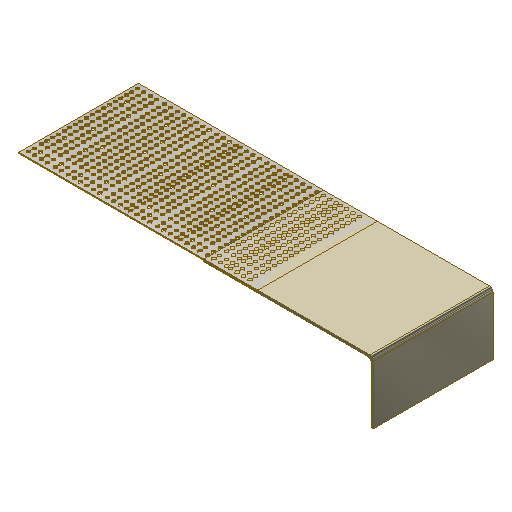
# Autodesk Inventor part: eletrodo - nickel e titanio
Saved by Autodesk Inventor 2025 (Build 290162000, 162)
## iProperties
Created: 2024-12-11
Part Number: eletrodo - nickel e titanio
Material: Genérico
Document SubType Name: Modeling
Designer: November
Density: 1 g/cm^3
Appearance: Padrão
Author: November
Autodesk Inventor part; units mm, degrees
(part 1 of 4)
ref_plane "YZ Plane" through (0, 0, 0) normal (1, 0, 0) x (0, 1, 0)
ref_plane "XZ Plane" through (0, 0, 0) normal (0, 1, 0) x (-1, 0, 0)
ref_plane "XY Plane" through (0, 0, 0) normal (0, 0, 1) x (1, 0, 0)
sketch "Esboço1" plane through (0, 0, 0) normal (0, 0, 1) x (1, 0, 0)
  line L0 (0, 0) -> (0, 5)
  line L1 (0, 5) -> (-14, 5)
  line L2 (0, 0) -> (0.2, 0)
  line L3 (0.2, 0) -> (0.2, 5.2)
  line L4 (-14, 5) -> (-14, 5.2)
  line L5 (-14, 5.2) -> (0.2, 5.2)
  dimension "d0" = 5
  dimension "d1" = 14
  dimension "d2" = 0.2
  dimension "d3" = 5.2
  dimension "d4" = 0.2
  constraints: 12 end point, 2 horizontal, 2 perpendicular, 2 vertical, 1 point on line
  measures "d0" distance of L0.start L0.end
  measures "d1" distance of L0.end L1.end
  measures "d2" distance of L0.start L2.end
  measures "d3" distance of L2.end L3.end
  measures "d4" distance of L1.end L4.end
extrude "Extrusão1" add sketch "Esboço1" along normal blind 10
fillet "Arredondamento1" radius 0.3 1 edges at (0.2, 5.2, 5)
fillet "Arredondamento2" radius 0.3 1 edges at (0, 5, 5)
sketch "Esboço2" plane through (-14, 5.2, 10) normal (0, 1, 0) x (1, 0, 0)
  line L0 (0, 10) -> (13.7, 10)
  line L1 (4.5193, 10) -> (-15.4807, 10)
  line L2 (-15.4807, 10) -> (-15.4807, 0)
  line L3 (-15.4807, 0) -> (4.5193, 0)
  line L4 (4.5193, 0) -> (4.5193, 10)
  point P0 (14, 10)
  point P1 (-5.4807, 0)
  dimension "d9" = 20
  dimension "d10" = 10
  constraints: 8 end point, 2 parallel, 1 horizontal, 1 midpoint, 1 perpendicular, 1 point on line
  measures "d9" distance of L3.end L2.end
  measures "d10" distance from line of point (-5.481, 0) L1
extrude "Extrusão2" add sketch "Esboço2" against normal blind 0.1 separate body
sketch "Esboço3" plane through (-14, 5.2, 10) normal (0, 1, 0) x (1, 0, 0)
  line L0 (-15.1346, 9.764) -> (-15.3015, 9.5833)
  line L1 (-15.3015, 9.5833) -> (-15.1346, 9.3971)
  line L2 (-15.1346, 9.764) -> (-14.9676, 9.5833)
  line L3 (-14.9676, 9.5833) -> (-15.1346, 9.3971)
  line L4 (-15.1346, 9.2863) -> (-15.3015, 9.1056)
  line L5 (-15.3015, 9.1056) -> (-15.1346, 8.9195)
  line L6 (-15.1346, 9.2863) -> (-14.9676, 9.1056)
  line L7 (-14.9676, 9.1056) -> (-15.1346, 8.9195)
  line L8 (-15.1346, 8.827) -> (-15.3015, 8.6463)
  line L9 (-15.3015, 8.6463) -> (-15.1346, 8.4602)
  line L10 (-15.1346, 8.827) -> (-14.9676, 8.6463)
  line L11 (-14.9676, 8.6463) -> (-15.1346, 8.4602)
  line L12 (-15.1346, 8.3637) -> (-15.3015, 8.183)
  line L13 (-15.3015, 8.183) -> (-15.1346, 7.9969)
  line L14 (-15.1346, 8.3637) -> (-14.9676, 8.183)
  line L15 (-14.9676, 8.183) -> (-15.1346, 7.9969)
  line L16 (-15.1346, 7.8983) -> (-15.3015, 7.7177)
  line L17 (-15.3015, 7.7177) -> (-15.1346, 7.5315)
  line L18 (-15.1346, 7.8983) -> (-14.9676, 7.7177)
  line L19 (-14.9676, 7.7177) -> (-15.1346, 7.5315)
  line L20 (-15.1346, 7.4088) -> (-15.3015, 7.2281)
  line L21 (-15.3015, 7.2281) -> (-15.1346, 7.042)
  line L22 (-15.1346, 7.4088) -> (-14.9676, 7.2281)
  line L23 (-14.9676, 7.2281) -> (-15.1346, 7.042)
  line L24 (-15.1346, 6.9434) -> (-15.3015, 6.7628)
  line L25 (-15.3015, 6.7628) -> (-15.1346, 6.5766)
  line L26 (-15.1346, 6.9434) -> (-14.9676, 6.7628)
  line L27 (-14.9676, 6.7628) -> (-15.1346, 6.5766)
  line L28 (-15.1346, 6.4539) -> (-15.3015, 6.2732)
  line L29 (-15.3015, 6.2732) -> (-15.1346, 6.0871)
  line L30 (-15.1346, 6.4539) -> (-14.9676, 6.2732)
  line L31 (-14.9676, 6.2732) -> (-15.1346, 6.0871)
  line L32 (-15.1346, 5.9825) -> (-15.3015, 5.8018)
  line L33 (-15.3015, 5.8018) -> (-15.1346, 5.6157)
  line L34 (-15.1346, 5.9825) -> (-14.9676, 5.8018)
  line L35 (-14.9676, 5.8018) -> (-15.1346, 5.6157)
  line L36 (-15.1346, 5.4909) -> (-15.3015, 5.3102)
  line L37 (-15.3015, 5.3102) -> (-15.1346, 5.124)
  line L38 (-15.1346, 5.4909) -> (-14.9676, 5.3102)
  line L39 (-14.9676, 5.3102) -> (-15.1346, 5.124)
  line L40 (-15.1346, 5.0132) -> (-15.3015, 4.8325)
  line L41 (-15.3015, 4.8325) -> (-15.1346, 4.6463)
  line L42 (-15.1346, 5.0132) -> (-14.9676, 4.8325)
  line L43 (-14.9676, 4.8325) -> (-15.1346, 4.6463)
  line L44 (-15.1346, 4.5539) -> (-15.3015, 4.3732)
  line L45 (-15.3015, 4.3732) -> (-15.1346, 4.187)
  line L46 (-15.1346, 4.5539) -> (-14.9676, 4.3732)
  line L47 (-14.9676, 4.3732) -> (-15.1346, 4.187)
  line L48 (-15.1346, 4.0906) -> (-15.3015, 3.9099)
  line L49 (-15.3015, 3.9099) -> (-15.1346, 3.7237)
  line L50 (-15.1346, 4.0906) -> (-14.9676, 3.9099)
  line L51 (-14.9676, 3.9099) -> (-15.1346, 3.7237)
  line L52 (-15.1346, 3.6252) -> (-15.3015, 3.4445)
  line L53 (-15.3015, 3.4445) -> (-15.1346, 3.2584)
  line L54 (-15.1346, 3.6252) -> (-14.9676, 3.4445)
  line L55 (-14.9676, 3.4445) -> (-15.1346, 3.2584)
  line L56 (-15.1346, 3.1357) -> (-15.3015, 2.955)
  line L57 (-15.3015, 2.955) -> (-15.1346, 2.7688)
  line L58 (-15.1346, 3.1357) -> (-14.9676, 2.955)
  line L59 (-14.9676, 2.955) -> (-15.1346, 2.7688)
  line L60 (-15.1346, 2.6703) -> (-15.3015, 2.4896)
  line L61 (-15.3015, 2.4896) -> (-15.1346, 2.3035)
  line L62 (-15.1346, 2.6703) -> (-14.9676, 2.4896)
  line L63 (-14.9676, 2.4896) -> (-15.1346, 2.3035)
  line L64 (-15.1346, 2.1808) -> (-15.3015, 2.0001)
  line L65 (-15.3015, 2.0001) -> (-15.1346, 1.8139)
  line L66 (-15.1346, 2.1808) -> (-14.9676, 2.0001)
  line L67 (-14.9676, 2.0001) -> (-15.1346, 1.8139)
  line L68 (-15.1346, 1.7094) -> (-15.3015, 1.5287)
  line L69 (-15.3015, 1.5287) -> (-15.1346, 1.3425)
  line L70 (-15.1346, 1.7094) -> (-14.9676, 1.5287)
  line L71 (-14.9676, 1.5287) -> (-15.1346, 1.3425)
  line L72 (-15.1346, 1.1085) -> (-15.3015, 0.9278)
  line L73 (-15.3015, 0.9278) -> (-15.1346, 0.7417)
  line L74 (-15.1346, 1.1085) -> (-14.9676, 0.9278)
  line L75 (-14.9676, 0.9278) -> (-15.1346, 0.7417)
  line L76 (-15.1346, 0.6309) -> (-15.3015, 0.4502)
  line L77 (-15.3015, 0.4502) -> (-15.1346, 0.264)
  line L78 (-15.1346, 0.6309) -> (-14.9676, 0.4502)
  line L79 (-14.9676, 0.4502) -> (-15.1346, 0.264)
  line L80 (-14.6177, 9.764) -> (-14.7847, 9.5833)
  line L81 (-14.7847, 9.5833) -> (-14.6177, 9.3971)
  line L82 (-14.6177, 9.764) -> (-14.4507, 9.5833)
  line L83 (-14.4507, 9.5833) -> (-14.6177, 9.3971)
  line L84 (-14.6177, 9.2863) -> (-14.7847, 9.1056)
  line L85 (-14.7847, 9.1056) -> (-14.6177, 8.9195)
  line L86 (-14.6177, 9.2863) -> (-14.4507, 9.1056)
  line L87 (-14.4507, 9.1056) -> (-14.6177, 8.9195)
  line L88 (-14.6177, 8.827) -> (-14.7847, 8.6463)
  line L89 (-14.7847, 8.6463) -> (-14.6177, 8.4602)
  line L90 (-14.6177, 8.827) -> (-14.4507, 8.6463)
  line L91 (-14.4507, 8.6463) -> (-14.6177, 8.4602)
  line L92 (-14.6177, 8.3637) -> (-14.7847, 8.183)
  line L93 (-14.7847, 8.183) -> (-14.6177, 7.9969)
  line L94 (-14.6177, 8.3637) -> (-14.4507, 8.183)
  line L95 (-14.4507, 8.183) -> (-14.6177, 7.9969)
  line L96 (-14.6177, 7.8983) -> (-14.7847, 7.7177)
  line L97 (-14.7847, 7.7177) -> (-14.6177, 7.5315)
  line L98 (-14.6177, 7.8983) -> (-14.4507, 7.7177)
  line L99 (-14.4507, 7.7177) -> (-14.6177, 7.5315)
  line L100 (-14.6177, 7.4088) -> (-14.7847, 7.2281)
  line L101 (-14.7847, 7.2281) -> (-14.6177, 7.042)
  line L102 (-14.6177, 7.4088) -> (-14.4507, 7.2281)
  line L103 (-14.4507, 7.2281) -> (-14.6177, 7.042)
  line L104 (-14.6177, 6.9434) -> (-14.7847, 6.7628)
  line L105 (-14.7847, 6.7628) -> (-14.6177, 6.5766)
  line L106 (-14.6177, 6.9434) -> (-14.4507, 6.7628)
  line L107 (-14.4507, 6.7628) -> (-14.6177, 6.5766)
  line L108 (-14.6177, 6.4539) -> (-14.7847, 6.2732)
  line L109 (-14.7847, 6.2732) -> (-14.6177, 6.0871)
  line L110 (-14.6177, 6.4539) -> (-14.4507, 6.2732)
  line L111 (-14.4507, 6.2732) -> (-14.6177, 6.0871)
  line L112 (-14.6177, 5.9825) -> (-14.7847, 5.8018)
  line L113 (-14.7847, 5.8018) -> (-14.6177, 5.6157)
  line L114 (-14.6177, 5.9825) -> (-14.4507, 5.8018)
  line L115 (-14.4507, 5.8018) -> (-14.6177, 5.6157)
  line L116 (-14.6177, 5.4909) -> (-14.7847, 5.3102)
  line L117 (-14.7847, 5.3102) -> (-14.6177, 5.124)
  line L118 (-14.6177, 5.4909) -> (-14.4507, 5.3102)
  line L119 (-14.6177, 4.5539) -> (-14.7847, 4.3732)
  line L120 (-14.6177, 4.5539) -> (-14.4507, 4.3732)
  line L121 (-14.7847, 4.8325) -> (-14.6177, 4.6463)
  line L122 (-14.4507, 4.8325) -> (-14.6177, 4.6463)
  line L123 (-14.6177, 5.0132) -> (-14.4507, 4.8325)
  line L124 (-14.4507, 5.3102) -> (-14.6177, 5.124)
  line L125 (-14.6177, 5.0132) -> (-14.7847, 4.8325)
  line L126 (-14.7847, 4.3732) -> (-14.6177, 4.187)
  line L127 (-14.4507, 4.3732) -> (-14.6177, 4.187)
  line L128 (-14.6177, 4.0906) -> (-14.7847, 3.9099)
  line L129 (-14.6177, 4.0906) -> (-14.4507, 3.9099)
  line L130 (-14.7847, 3.9099) -> (-14.6177, 3.7237)
  line L131 (-14.4507, 3.9099) -> (-14.6177, 3.7237)
  line L132 (-14.6177, 3.6252) -> (-14.7847, 3.4445)
  line L133 (-14.6177, 3.6252) -> (-14.4507, 3.4445)
  line L134 (-14.7847, 3.4445) -> (-14.6177, 3.2584)
  line L135 (-14.4507, 3.4445) -> (-14.6177, 3.2584)
  line L136 (-14.6177, 3.1357) -> (-14.7847, 2.955)
  line L137 (-14.6177, 3.1357) -> (-14.4507, 2.955)
  line L138 (-14.7847, 2.955) -> (-14.6177, 2.7688)
  line L139 (-14.4507, 2.955) -> (-14.6177, 2.7688)
  line L140 (-14.6177, 2.6703) -> (-14.4507, 2.4896)
  line L141 (-14.6177, 2.6703) -> (-14.7847, 2.4896)
  line L142 (-14.4507, 2.4896) -> (-14.6177, 2.3035)
  line L143 (-14.7847, 2.4896) -> (-14.6177, 2.3035)
  line L144 (-14.6177, 2.1808) -> (-14.7847, 2.0001)
  line L145 (-14.6177, 2.1808) -> (-14.4507, 2.0001)
  line L146 (-14.7847, 2.0001) -> (-14.6177, 1.8139)
  line L147 (-14.4507, 2.0001) -> (-14.6177, 1.8139)
  line L148 (-14.6177, 1.7094) -> (-14.7847, 1.5287)
  line L149 (-14.6177, 1.7094) -> (-14.4507, 1.5287)
  line L150 (-14.7847, 1.5287) -> (-14.6177, 1.3425)
  line L151 (-14.4507, 1.5287) -> (-14.6177, 1.3425)
  line L152 (-14.6177, 1.1085) -> (-14.7847, 0.9278)
  line L153 (-14.7847, 0.9278) -> (-14.6177, 0.7417)
  line L154 (-14.6177, 1.1085) -> (-14.4507, 0.9278)
  line L155 (-14.7847, 0.4502) -> (-14.6177, 0.264)
  line L156 (-14.4507, 0.4502) -> (-14.6177, 0.264)
  line L157 (-14.6177, 0.6309) -> (-14.4507, 0.4502)
  line L158 (-14.4507, 0.9278) -> (-14.6177, 0.7417)
  line L159 (-14.6177, 0.6309) -> (-14.7847, 0.4502)
  line L160 (-14.0508, 9.764) -> (-14.2178, 9.5833)
  line L161 (-14.2178, 9.5833) -> (-14.0508, 9.3971)
  line L162 (-14.0508, 9.764) -> (-13.8838, 9.5833)
  line L163 (-13.8838, 9.5833) -> (-14.0508, 9.3971)
  line L164 (-14.0508, 9.2863) -> (-14.2178, 9.1056)
  line L165 (-14.2178, 9.1056) -> (-14.0508, 8.9195)
  line L166 (-14.0508, 9.2863) -> (-13.8838, 9.1056)
  line L167 (-13.8838, 9.1056) -> (-14.0508, 8.9195)
  line L168 (-14.0508, 8.827) -> (-14.2178, 8.6463)
  line L169 (-14.2178, 8.6463) -> (-14.0508, 8.4602)
  line L170 (-14.0508, 8.827) -> (-13.8838, 8.6463)
  line L171 (-13.8838, 8.6463) -> (-14.0508, 8.4602)
  line L172 (-14.0508, 8.3637) -> (-14.2178, 8.183)
  line L173 (-14.2178, 8.183) -> (-14.0508, 7.9969)
  line L174 (-14.0508, 8.3637) -> (-13.8838, 8.183)
  line L175 (-13.8838, 8.183) -> (-14.0508, 7.9969)
  line L176 (-14.0508, 7.8983) -> (-14.2178, 7.7177)
  line L177 (-14.2178, 7.7177) -> (-14.0508, 7.5315)
  line L178 (-14.0508, 7.8983) -> (-13.8838, 7.7177)
  line L179 (-13.8838, 7.7177) -> (-14.0508, 7.5315)
  line L180 (-14.0508, 7.4088) -> (-14.2178, 7.2281)
  line L181 (-14.2178, 7.2281) -> (-14.0508, 7.042)
  line L182 (-14.0508, 7.4088) -> (-13.8838, 7.2281)
  line L183 (-13.8838, 7.2281) -> (-14.0508, 7.042)
  line L184 (-14.0508, 6.9434) -> (-14.2178, 6.7628)
  line L185 (-14.2178, 6.7628) -> (-14.0508, 6.5766)
  line L186 (-14.0508, 6.9434) -> (-13.8838, 6.7628)
  line L187 (-13.8838, 6.7628) -> (-14.0508, 6.5766)
  line L188 (-14.0508, 6.4539) -> (-14.2178, 6.2732)
  line L189 (-14.2178, 6.2732) -> (-14.0508, 6.0871)
  line L190 (-14.0508, 6.4539) -> (-13.8838, 6.2732)
  line L191 (-13.8838, 6.2732) -> (-14.0508, 6.0871)
  line L192 (-14.0508, 5.9825) -> (-14.2178, 5.8018)
  line L193 (-14.2178, 5.8018) -> (-14.0508, 5.6157)
  line L194 (-14.0508, 5.9825) -> (-13.8838, 5.8018)
  line L195 (-13.8838, 5.8018) -> (-14.0508, 5.6157)
  line L196 (-14.0508, 5.4909) -> (-14.2178, 5.3102)
  line L197 (-14.2178, 5.3102) -> (-14.0508, 5.124)
  line L198 (-14.0508, 5.4909) -> (-13.8838, 5.3102)
  line L199 (-14.0508, 4.5539) -> (-14.2178, 4.3732)
  line L200 (-14.0508, 4.5539) -> (-13.8838, 4.3732)
  line L201 (-14.2178, 4.8325) -> (-14.0508, 4.6463)
  line L202 (-13.8838, 4.8325) -> (-14.0508, 4.6463)
  line L203 (-14.0508, 5.0132) -> (-13.8838, 4.8325)
  line L204 (-13.8838, 5.3102) -> (-14.0508, 5.124)
  line L205 (-14.0508, 5.0132) -> (-14.2178, 4.8325)
  line L206 (-14.2178, 4.3732) -> (-14.0508, 4.187)
  line L207 (-13.8838, 4.3732) -> (-14.0508, 4.187)
  line L208 (-14.0508, 4.0906) -> (-14.2178, 3.9099)
  line L209 (-14.0508, 4.0906) -> (-13.8838, 3.9099)
  line L210 (-14.2178, 3.9099) -> (-14.0508, 3.7237)
  line L211 (-13.8838, 3.9099) -> (-14.0508, 3.7237)
  line L212 (-14.0508, 3.6252) -> (-14.2178, 3.4445)
  line L213 (-14.0508, 3.6252) -> (-13.8838, 3.4445)
  line L214 (-14.2178, 3.4445) -> (-14.0508, 3.2584)
  line L215 (-13.8838, 3.4445) -> (-14.0508, 3.2584)
  line L216 (-14.0508, 3.1357) -> (-14.2178, 2.955)
  line L217 (-14.0508, 3.1357) -> (-13.8838, 2.955)
  line L218 (-14.2178, 2.955) -> (-14.0508, 2.7688)
  line L219 (-13.8838, 2.955) -> (-14.0508, 2.7688)
  line L220 (-14.0508, 2.6703) -> (-13.8838, 2.4896)
  line L221 (-14.0508, 2.6703) -> (-14.2178, 2.4896)
  line L222 (-13.8838, 2.4896) -> (-14.0508, 2.3035)
  line L223 (-14.2178, 2.4896) -> (-14.0508, 2.3035)
  line L224 (-14.0508, 2.1808) -> (-14.2178, 2.0001)
  line L225 (-14.0508, 2.1808) -> (-13.8838, 2.0001)
  line L226 (-14.2178, 2.0001) -> (-14.0508, 1.8139)
  line L227 (-13.8838, 2.0001) -> (-14.0508, 1.8139)
  line L228 (-14.0508, 1.7094) -> (-14.2178, 1.5287)
  line L229 (-14.0508, 1.7094) -> (-13.8838, 1.5287)
  line L230 (-14.2178, 1.5287) -> (-14.0508, 1.3425)
  line L231 (-13.8838, 1.5287) -> (-14.0508, 1.3425)
  line L232 (-14.0508, 1.1085) -> (-14.2178, 0.9278)
  line L233 (-14.2178, 0.9278) -> (-14.0508, 0.7417)
  line L234 (-14.0508, 1.1085) -> (-13.8838, 0.9278)
  line L235 (-14.2178, 0.4502) -> (-14.0508, 0.264)
  line L236 (-13.8838, 0.4502) -> (-14.0508, 0.264)
  line L237 (-14.0508, 0.6309) -> (-13.8838, 0.4502)
  line L238 (-13.8838, 0.9278) -> (-14.0508, 0.7417)
  line L239 (-14.0508, 0.6309) -> (-14.2178, 0.4502)
  line L240 (-13.534, 9.764) -> (-13.701, 9.5833)
  line L241 (-13.701, 9.5833) -> (-13.534, 9.3971)
  line L242 (-13.534, 9.764) -> (-13.367, 9.5833)
  line L243 (-13.534, 8.827) -> (-13.701, 8.6463)
  line L244 (-13.534, 8.827) -> (-13.367, 8.6463)
  line L245 (-13.367, 9.1056) -> (-13.534, 8.9195)
  line L246 (-13.534, 9.2863) -> (-13.701, 9.1056)
  line L247 (-13.534, 9.2863) -> (-13.367, 9.1056)
  line L248 (-13.367, 9.5833) -> (-13.534, 9.3971)
  line L249 (-13.701, 9.1056) -> (-13.534, 8.9195)
  line L250 (-13.701, 8.6463) -> (-13.534, 8.4602)
  line L251 (-13.367, 8.6463) -> (-13.534, 8.4602)
  line L252 (-13.534, 8.3637) -> (-13.701, 8.183)
  line L253 (-13.534, 8.3637) -> (-13.367, 8.183)
  line L254 (-13.701, 8.183) -> (-13.534, 7.9969)
  line L255 (-13.367, 8.183) -> (-13.534, 7.9969)
  line L256 (-13.534, 7.8983) -> (-13.701, 7.7177)
  line L257 (-13.701, 7.7177) -> (-13.534, 7.5315)
  line L258 (-13.367, 7.7177) -> (-13.534, 7.5315)
  line L259 (-13.534, 7.8983) -> (-13.367, 7.7177)
  line L260 (-13.534, 7.4088) -> (-13.367, 7.2281)
  line L261 (-13.534, 7.4088) -> (-13.701, 7.2281)
  line L262 (-13.701, 7.2281) -> (-13.534, 7.042)
  line L263 (-13.367, 7.2281) -> (-13.534, 7.042)
  line L264 (-13.534, 6.9434) -> (-13.367, 6.7628)
  line L265 (-13.367, 6.7628) -> (-13.534, 6.5766)
  line L266 (-13.701, 6.7628) -> (-13.534, 6.5766)
  line L267 (-13.534, 6.9434) -> (-13.701, 6.7628)
  line L268 (-13.534, 6.4539) -> (-13.701, 6.2732)
  line L269 (-13.534, 6.4539) -> (-13.367, 6.2732)
  line L270 (-13.701, 6.2732) -> (-13.534, 6.0871)
  line L271 (-13.367, 6.2732) -> (-13.534, 6.0871)
  line L272 (-13.534, 5.9825) -> (-13.701, 5.8018)
  line L273 (-13.534, 5.9825) -> (-13.367, 5.8018)
  line L274 (-13.701, 5.8018) -> (-13.534, 5.6157)
  line L275 (-13.367, 5.8018) -> (-13.534, 5.6157)
  line L276 (-13.534, 5.4909) -> (-13.701, 5.3102)
  line L277 (-13.534, 5.4909) -> (-13.367, 5.3102)
  line L278 (-13.701, 5.3102) -> (-13.534, 5.124)
  line L279 (-13.367, 5.3102) -> (-13.534, 5.124)
  line L280 (-13.534, 5.0132) -> (-13.701, 4.8325)
  line L281 (-13.534, 5.0132) -> (-13.367, 4.8325)
  line L282 (-13.701, 4.8325) -> (-13.534, 4.6463)
  line L283 (-13.367, 4.8325) -> (-13.534, 4.6463)
  line L284 (-13.534, 4.5539) -> (-13.367, 4.3732)
  line L285 (-13.534, 4.5539) -> (-13.701, 4.3732)
  line L286 (-13.701, 4.3732) -> (-13.534, 4.187)
  line L287 (-13.367, 4.3732) -> (-13.534, 4.187)
  line L288 (-13.534, 4.0906) -> (-13.701, 3.9099)
  line L289 (-13.534, 4.0906) -> (-13.367, 3.9099)
  line L290 (-13.701, 3.9099) -> (-13.534, 3.7237)
  line L291 (-13.367, 3.9099) -> (-13.534, 3.7237)
  line L292 (-13.534, 3.6252) -> (-13.701, 3.4445)
  line L293 (-13.534, 3.6252) -> (-13.367, 3.4445)
  line L294 (-13.701, 3.4445) -> (-13.534, 3.2584)
  line L295 (-13.367, 3.4445) -> (-13.534, 3.2584)
  line L296 (-13.534, 3.1357) -> (-13.701, 2.955)
  line L297 (-13.534, 3.1357) -> (-13.367, 2.955)
  line L298 (-13.701, 2.955) -> (-13.534, 2.7688)
  line L299 (-13.367, 2.955) -> (-13.534, 2.7688)
  line L300 (-13.534, 2.6703) -> (-13.367, 2.4896)
  line L301 (-13.534, 2.6703) -> (-13.701, 2.4896)
  line L302 (-13.701, 2.4896) -> (-13.534, 2.3035)
  line L303 (-13.367, 2.4896) -> (-13.534, 2.3035)
  line L304 (-13.534, 1.1085) -> (-13.701, 0.9278)
  line L305 (-13.534, 1.1085) -> (-13.367, 0.9278)
  line L306 (-13.701, 0.9278) -> (-13.534, 0.7417)
  line L307 (-13.534, 0.6309) -> (-13.367, 0.4502)
  line L308 (-13.534, 0.6309) -> (-13.701, 0.4502)
  line L309 (-13.701, 0.4502) -> (-13.534, 0.264)
  line L310 (-13.367, 0.4502) -> (-13.534, 0.264)
  line L311 (-13.367, 0.9278) -> (-13.534, 0.7417)
  line L312 (-13.534, 2.1808) -> (-13.367, 2.0001)
  line L313 (-13.534, 2.1808) -> (-13.701, 2.0001)
  line L314 (-13.701, 2.0001) -> (-13.534, 1.8139)
  line L315 (-13.367, 2.0001) -> (-13.534, 1.8139)
  line L316 (-13.534, 1.7094) -> (-13.367, 1.5287)
  line L317 (-13.534, 1.7094) -> (-13.701, 1.5287)
  line L318 (-13.367, 1.5287) -> (-13.534, 1.3425)
  line L319 (-13.701, 1.5287) -> (-13.534, 1.3425)
  line L320 (-12.8812, 9.764) -> (-13.0482, 9.5833)
  line L321 (-13.0482, 9.5833) -> (-12.8812, 9.3971)
  line L322 (-12.8812, 9.764) -> (-12.7142, 9.5833)
  line L323 (-12.7142, 9.5833) -> (-12.8812, 9.3971)
  line L324 (-12.8812, 9.2863) -> (-13.0482, 9.1056)
  line L325 (-13.0482, 9.1056) -> (-12.8812, 8.9195)
  line L326 (-12.8812, 9.2863) -> (-12.7142, 9.1056)
  line L327 (-12.7142, 9.1056) -> (-12.8812, 8.9195)
  line L328 (-12.8812, 8.827) -> (-13.0482, 8.6463)
  line L329 (-13.0482, 8.6463) -> (-12.8812, 8.4602)
  line L330 (-12.8812, 8.827) -> (-12.7142, 8.6463)
  line L331 (-12.7142, 8.6463) -> (-12.8812, 8.4602)
  line L332 (-12.8812, 8.3637) -> (-13.0482, 8.183)
  line L333 (-13.0482, 8.183) -> (-12.8812, 7.9969)
  line L334 (-12.8812, 8.3637) -> (-12.7142, 8.183)
  line L335 (-12.7142, 8.183) -> (-12.8812, 7.9969)
  line L336 (-12.8812, 7.8983) -> (-13.0482, 7.7177)
  line L337 (-13.0482, 7.7177) -> (-12.8812, 7.5315)
  line L338 (-12.8812, 7.8983) -> (-12.7142, 7.7177)
  line L339 (-12.7142, 7.7177) -> (-12.8812, 7.5315)
  line L340 (-12.8812, 7.4088) -> (-13.0482, 7.2281)
  line L341 (-13.0482, 7.2281) -> (-12.8812, 7.042)
  line L342 (-12.8812, 7.4088) -> (-12.7142, 7.2281)
  line L343 (-12.7142, 7.2281) -> (-12.8812, 7.042)
  line L344 (-12.8812, 6.9434) -> (-13.0482, 6.7628)
  line L345 (-13.0482, 6.7628) -> (-12.8812, 6.5766)
  line L346 (-12.8812, 6.9434) -> (-12.7142, 6.7628)
  line L347 (-12.7142, 6.7628) -> (-12.8812, 6.5766)
  line L348 (-12.8812, 6.4539) -> (-13.0482, 6.2732)
  line L349 (-13.0482, 6.2732) -> (-12.8812, 6.0871)
  line L350 (-12.8812, 6.4539) -> (-12.7142, 6.2732)
  line L351 (-12.7142, 6.2732) -> (-12.8812, 6.0871)
  line L352 (-12.8812, 5.9825) -> (-13.0482, 5.8018)
  line L353 (-13.0482, 5.8018) -> (-12.8812, 5.6157)
  line L354 (-12.8812, 5.9825) -> (-12.7142, 5.8018)
  line L355 (-12.7142, 5.8018) -> (-12.8812, 5.6157)
  line L356 (-12.8812, 5.4909) -> (-13.0482, 5.3102)
  line L357 (-13.0482, 5.3102) -> (-12.8812, 5.124)
  line L358 (-12.8812, 5.4909) -> (-12.7142, 5.3102)
  line L359 (-12.8812, 4.5539) -> (-13.0482, 4.3732)
  line L360 (-12.8812, 4.5539) -> (-12.7142, 4.3732)
  line L361 (-13.0482, 4.8325) -> (-12.8812, 4.6463)
  line L362 (-12.7142, 4.8325) -> (-12.8812, 4.6463)
  line L363 (-12.8812, 5.0132) -> (-12.7142, 4.8325)
  line L364 (-12.7142, 5.3102) -> (-12.8812, 5.124)
  line L365 (-12.8812, 5.0132) -> (-13.0482, 4.8325)
  line L366 (-13.0482, 4.3732) -> (-12.8812, 4.187)
  line L367 (-12.7142, 4.3732) -> (-12.8812, 4.187)
  line L368 (-12.8812, 4.0906) -> (-13.0482, 3.9099)
  line L369 (-12.8812, 4.0906) -> (-12.7142, 3.9099)
  line L370 (-13.0482, 3.9099) -> (-12.8812, 3.7237)
  line L371 (-12.7142, 3.9099) -> (-12.8812, 3.7237)
  line L372 (-12.8812, 3.6252) -> (-13.0482, 3.4445)
  line L373 (-12.8812, 3.6252) -> (-12.7142, 3.4445)
  line L374 (-13.0482, 3.4445) -> (-12.8812, 3.2584)
  line L375 (-12.7142, 3.4445) -> (-12.8812, 3.2584)
  line L376 (-12.8812, 3.1357) -> (-13.0482, 2.955)
  line L377 (-12.8812, 3.1357) -> (-12.7142, 2.955)
  line L378 (-13.0482, 2.955) -> (-12.8812, 2.7688)
  line L379 (-12.7142, 2.955) -> (-12.8812, 2.7688)
  line L380 (-12.8812, 2.6703) -> (-12.7142, 2.4896)
  line L381 (-12.8812, 2.6703) -> (-13.0482, 2.4896)
  line L382 (-12.7142, 2.4896) -> (-12.8812, 2.3035)
  line L383 (-13.0482, 2.4896) -> (-12.8812, 2.3035)
  line L384 (-12.8812, 2.1808) -> (-13.0482, 2.0001)
  line L385 (-12.8812, 2.1808) -> (-12.7142, 2.0001)
  line L386 (-13.0482, 2.0001) -> (-12.8812, 1.8139)
  line L387 (-12.7142, 2.0001) -> (-12.8812, 1.8139)
  line L388 (-12.8812, 1.7094) -> (-13.0482, 1.5287)
  line L389 (-12.8812, 1.7094) -> (-12.7142, 1.5287)
  line L390 (-13.0482, 1.5287) -> (-12.8812, 1.3425)
  line L391 (-12.7142, 1.5287) -> (-12.8812, 1.3425)
  line L392 (-12.8812, 1.1085) -> (-13.0482, 0.9278)
  line L393 (-13.0482, 0.9278) -> (-12.8812, 0.7417)
  line L394 (-12.8812, 1.1085) -> (-12.7142, 0.9278)
  line L395 (-13.0482, 0.4502) -> (-12.8812, 0.264)
  line L396 (-12.7142, 0.4502) -> (-12.8812, 0.264)
  line L397 (-12.8812, 0.6309) -> (-12.7142, 0.4502)
  line L398 (-12.7142, 0.9278) -> (-12.8812, 0.7417)
  line L399 (-12.8812, 0.6309) -> (-13.0482, 0.4502)
  line L400 (-12.3644, 9.764) -> (-12.5314, 9.5833)
  line L401 (-12.5314, 9.5833) -> (-12.3644, 9.3971)
  line L402 (-12.3644, 9.764) -> (-12.1974, 9.5833)
  line L403 (-12.3644, 8.827) -> (-12.5314, 8.6463)
  line L404 (-12.3644, 8.827) -> (-12.1974, 8.6463)
  line L405 (-12.1974, 9.1056) -> (-12.3644, 8.9195)
  line L406 (-12.3644, 9.2863) -> (-12.5314, 9.1056)
  line L407 (-12.3644, 9.2863) -> (-12.1974, 9.1056)
  line L408 (-12.1974, 9.5833) -> (-12.3644, 9.3971)
  line L409 (-12.5314, 9.1056) -> (-12.3644, 8.9195)
  line L410 (-12.5314, 8.6463) -> (-12.3644, 8.4602)
  line L411 (-12.1974, 8.6463) -> (-12.3644, 8.4602)
  line L412 (-12.3644, 8.3637) -> (-12.5314, 8.183)
  line L413 (-12.3644, 8.3637) -> (-12.1974, 8.183)
  line L414 (-12.5314, 8.183) -> (-12.3644, 7.9969)
  line L415 (-12.1974, 8.183) -> (-12.3644, 7.9969)
  line L416 (-12.3644, 7.8983) -> (-12.5314, 7.7177)
  line L417 (-12.5314, 7.7177) -> (-12.3644, 7.5315)
  line L418 (-12.1974, 7.7177) -> (-12.3644, 7.5315)
  line L419 (-12.3644, 7.8983) -> (-12.1974, 7.7177)
  line L420 (-12.3644, 7.4088) -> (-12.1974, 7.2281)
  line L421 (-12.3644, 7.4088) -> (-12.5314, 7.2281)
  line L422 (-12.5314, 7.2281) -> (-12.3644, 7.042)
  line L423 (-12.1974, 7.2281) -> (-12.3644, 7.042)
  line L424 (-12.3644, 6.9434) -> (-12.1974, 6.7628)
  line L425 (-12.1974, 6.7628) -> (-12.3644, 6.5766)
  line L426 (-12.5314, 6.7628) -> (-12.3644, 6.5766)
  line L427 (-12.3644, 6.9434) -> (-12.5314, 6.7628)
  line L428 (-12.3644, 6.4539) -> (-12.5314, 6.2732)
  line L429 (-12.3644, 6.4539) -> (-12.1974, 6.2732)
  line L430 (-12.5314, 6.2732) -> (-12.3644, 6.0871)
  line L431 (-12.1974, 6.2732) -> (-12.3644, 6.0871)
  line L432 (-12.3644, 5.9825) -> (-12.5314, 5.8018)
  line L433 (-12.3644, 5.9825) -> (-12.1974, 5.8018)
  line L434 (-12.5314, 5.8018) -> (-12.3644, 5.6157)
  line L435 (-12.1974, 5.8018) -> (-12.3644, 5.6157)
  line L436 (-12.3644, 5.4909) -> (-12.5314, 5.3102)
  line L437 (-12.3644, 5.4909) -> (-12.1974, 5.3102)
  line L438 (-12.5314, 5.3102) -> (-12.3644, 5.124)
  line L439 (-12.1974, 5.3102) -> (-12.3644, 5.124)
  line L440 (-12.3644, 5.0132) -> (-12.5314, 4.8325)
  line L441 (-12.3644, 5.0132) -> (-12.1974, 4.8325)
  line L442 (-12.5314, 4.8325) -> (-12.3644, 4.6463)
  line L443 (-12.1974, 4.8325) -> (-12.3644, 4.6463)
  line L444 (-12.3644, 4.5539) -> (-12.1974, 4.3732)
  line L445 (-12.3644, 4.5539) -> (-12.5314, 4.3732)
  line L446 (-12.5314, 4.3732) -> (-12.3644, 4.187)
  line L447 (-12.1974, 4.3732) -> (-12.3644, 4.187)
  line L448 (-12.3644, 4.0906) -> (-12.5314, 3.9099)
  line L449 (-12.3644, 4.0906) -> (-12.1974, 3.9099)
  line L450 (-12.5314, 3.9099) -> (-12.3644, 3.7237)
  line L451 (-12.1974, 3.9099) -> (-12.3644, 3.7237)
  line L452 (-12.3644, 3.6252) -> (-12.5314, 3.4445)
  line L453 (-12.3644, 3.6252) -> (-12.1974, 3.4445)
  line L454 (-12.5314, 3.4445) -> (-12.3644, 3.2584)
  line L455 (-12.1974, 3.4445) -> (-12.3644, 3.2584)
  line L456 (-12.3644, 3.1357) -> (-12.5314, 2.955)
  line L457 (-12.3644, 3.1357) -> (-12.1974, 2.955)
  line L458 (-12.5314, 2.955) -> (-12.3644, 2.7688)
  line L459 (-12.1974, 2.955) -> (-12.3644, 2.7688)
  line L460 (-12.3644, 2.6703) -> (-12.1974, 2.4896)
  line L461 (-12.3644, 2.6703) -> (-12.5314, 2.4896)
  line L462 (-12.5314, 2.4896) -> (-12.3644, 2.3035)
  line L463 (-12.1974, 2.4896) -> (-12.3644, 2.3035)
  line L464 (-12.3644, 1.1085) -> (-12.5314, 0.9278)
  line L465 (-12.3644, 1.1085) -> (-12.1974, 0.9278)
  line L466 (-12.5314, 0.9278) -> (-12.3644, 0.7417)
  line L467 (-12.3644, 0.6309) -> (-12.1974, 0.4502)
  line L468 (-12.3644, 0.6309) -> (-12.5314, 0.4502)
  line L469 (-12.5314, 0.4502) -> (-12.3644, 0.264)
  line L470 (-12.1974, 0.4502) -> (-12.3644, 0.264)
  line L471 (-12.1974, 0.9278) -> (-12.3644, 0.7417)
  line L472 (-12.3644, 2.1808) -> (-12.1974, 2.0001)
  line L473 (-12.3644, 2.1808) -> (-12.5314, 2.0001)
  line L474 (-12.5314, 2.0001) -> (-12.3644, 1.8139)
  line L475 (-12.1974, 2.0001) -> (-12.3644, 1.8139)
  line L476 (-12.3644, 1.7094) -> (-12.1974, 1.5287)
  line L477 (-12.3644, 1.7094) -> (-12.5314, 1.5287)
  line L478 (-12.1974, 1.5287) -> (-12.3644, 1.3425)
  line L479 (-12.5314, 1.5287) -> (-12.3644, 1.3425)
  line L480 (-11.2807, 9.2863) -> (-11.4477, 9.1056)
  line L481 (-11.2807, 9.2863) -> (-11.1137, 9.1056)
  line L482 (-11.1137, 9.1056) -> (-11.2807, 8.9195)
  line L483 (-11.4477, 9.1056) -> (-11.2807, 8.9195)
  line L484 (-11.2807, 8.827) -> (-11.1137, 8.6463)
  line L485 (-11.2807, 8.827) -> (-11.4477, 8.6463)
  line L486 (-11.7975, 9.2863) -> (-11.6305, 9.1056)
  line L487 (-11.7975, 9.2863) -> (-11.9645, 9.1056)
  line L488 (-11.6305, 9.1056) -> (-11.7975, 8.9195)
  line L489 (-11.9645, 9.1056) -> (-11.7975, 8.9195)
  line L490 (-11.7975, 9.764) -> (-11.9645, 9.5833)
  line L491 (-11.9645, 9.5833) -> (-11.7975, 9.3971)
  line L492 (-11.6305, 9.5833) -> (-11.7975, 9.3971)
  line L493 (-11.7975, 9.764) -> (-11.6305, 9.5833)
  line L494 (-11.4477, 9.5833) -> (-11.2807, 9.3971)
  line L495 (-11.1137, 9.5833) -> (-11.2807, 9.3971)
  line L496 (-11.2807, 9.764) -> (-11.4477, 9.5833)
  line L497 (-11.2807, 9.764) -> (-11.1137, 9.5833)
  line L498 (-11.7975, 7.4088) -> (-11.9645, 7.2281)
  line L499 (-11.9645, 7.2281) -> (-11.7975, 7.042)
  line L500 (-11.7975, 6.4539) -> (-11.6305, 6.2732)
  line L501 (-11.7975, 6.4539) -> (-11.9645, 6.2732)
  line L502 (-11.6305, 6.2732) -> (-11.7975, 6.0871)
  line L503 (-11.9645, 6.2732) -> (-11.7975, 6.0871)
  line L504 (-11.2807, 5.9825) -> (-11.1137, 5.8018)
  line L505 (-11.2807, 5.9825) -> (-11.4477, 5.8018)
  line L506 (-11.1137, 5.8018) -> (-11.2807, 5.6157)
  line L507 (-11.4477, 5.8018) -> (-11.2807, 5.6157)
  line L508 (-11.7975, 5.9825) -> (-11.6305, 5.8018)
  line L509 (-11.7975, 5.9825) -> (-11.9645, 5.8018)
  line L510 (-11.6305, 5.8018) -> (-11.7975, 5.6157)
  line L511 (-11.9645, 5.8018) -> (-11.7975, 5.6157)
  line L512 (-11.4477, 4.8325) -> (-11.2807, 4.6463)
  line L513 (-11.1137, 4.8325) -> (-11.2807, 4.6463)
  line L514 (-11.7975, 5.0132) -> (-11.6305, 4.8325)
  line L515 (-11.7975, 5.0132) -> (-11.9645, 4.8325)
  line L516 (-11.2807, 4.5539) -> (-11.1137, 4.3732)
  line L517 (-11.2807, 4.5539) -> (-11.4477, 4.3732)
  line L518 (-11.6305, 4.8325) -> (-11.7975, 4.6463)
  line L519 (-11.9645, 4.8325) -> (-11.7975, 4.6463)
  line L520 (-11.7975, 4.5539) -> (-11.6305, 4.3732)
  line L521 (-11.7975, 4.5539) -> (-11.9645, 4.3732)
  line L522 (-11.6305, 3.4445) -> (-11.7975, 3.2584)
  line L523 (-11.9645, 3.4445) -> (-11.7975, 3.2584)
  line L524 (-11.7975, 3.6252) -> (-11.6305, 3.4445)
  line L525 (-11.7975, 3.6252) -> (-11.9645, 3.4445)
  line L526 (-11.9645, 3.9099) -> (-11.7975, 3.7237)
  line L527 (-11.7975, 4.0906) -> (-11.6305, 3.9099)
  line L528 (-11.7975, 4.0906) -> (-11.9645, 3.9099)
  line L529 (-11.6305, 3.9099) -> (-11.7975, 3.7237)
  line L530 (-11.7975, 8.827) -> (-11.9645, 8.6463)
  line L531 (-11.9645, 8.6463) -> (-11.7975, 8.4602)
  line L532 (-11.7975, 8.827) -> (-11.6305, 8.6463)
  line L533 (-11.6305, 8.6463) -> (-11.7975, 8.4602)
  line L534 (-11.7975, 8.3637) -> (-11.9645, 8.183)
  line L535 (-11.9645, 8.183) -> (-11.7975, 7.9969)
  line L536 (-11.7975, 8.3637) -> (-11.6305, 8.183)
  line L537 (-11.1137, 8.6463) -> (-11.2807, 8.4602)
  line L538 (-11.4477, 8.6463) -> (-11.2807, 8.4602)
  line L539 (-11.2807, 8.3637) -> (-11.1137, 8.183)
  line L540 (-11.1137, 8.183) -> (-11.2807, 7.9969)
  line L541 (-11.4477, 8.183) -> (-11.2807, 7.9969)
  line L542 (-11.6305, 8.183) -> (-11.7975, 7.9969)
  line L543 (-11.2807, 8.3637) -> (-11.4477, 8.183)
  line L544 (-11.7975, 7.8983) -> (-11.9645, 7.7177)
  line L545 (-11.9645, 7.7177) -> (-11.7975, 7.5315)
  line L546 (-11.7975, 7.4088) -> (-11.6305, 7.2281)
  line L547 (-11.6305, 7.2281) -> (-11.7975, 7.042)
  line L548 (-11.6305, 7.7177) -> (-11.7975, 7.5315)
  line L549 (-11.7975, 7.8983) -> (-11.6305, 7.7177)
  line L550 (-11.2807, 6.9434) -> (-11.4477, 6.7628)
  line L551 (-11.2807, 6.9434) -> (-11.1137, 6.7628)
  line L552 (-11.2807, 7.4088) -> (-11.4477, 7.2281)
  line L553 (-11.1137, 7.2281) -> (-11.2807, 7.042)
  line L554 (-11.4477, 7.7177) -> (-11.2807, 7.5315)
  line L555 (-11.2807, 7.8983) -> (-11.4477, 7.7177)
  line L556 (-11.2807, 7.8983) -> (-11.1137, 7.7177)
  line L557 (-11.1137, 7.7177) -> (-11.2807, 7.5315)
  line L558 (-11.2807, 7.4088) -> (-11.1137, 7.2281)
  line L559 (-11.4477, 7.2281) -> (-11.2807, 7.042)
  line L560 (-11.7975, 6.9434) -> (-11.9645, 6.7628)
  line L561 (-11.9645, 6.7628) -> (-11.7975, 6.5766)
  line L562 (-11.7975, 6.9434) -> (-11.6305, 6.7628)
  line L563 (-11.6305, 6.7628) -> (-11.7975, 6.5766)
  line L564 (-11.4477, 6.2732) -> (-11.2807, 6.0871)
  line L565 (-11.1137, 6.2732) -> (-11.2807, 6.0871)
  line L566 (-11.2807, 6.4539) -> (-11.4477, 6.2732)
  line L567 (-11.2807, 6.4539) -> (-11.1137, 6.2732)
  line L568 (-11.4477, 6.7628) -> (-11.2807, 6.5766)
  line L569 (-11.1137, 6.7628) -> (-11.2807, 6.5766)
  line L570 (-11.7975, 5.4909) -> (-11.9645, 5.3102)
  line L571 (-11.9645, 5.3102) -> (-11.7975, 5.124)
  line L572 (-11.7975, 5.4909) -> (-11.6305, 5.3102)
  line L573 (-11.2807, 5.0132) -> (-11.4477, 4.8325)
  line L574 (-11.6305, 5.3102) -> (-11.7975, 5.124)
  line L575 (-11.4477, 5.3102) -> (-11.2807, 5.124)
  line L576 (-11.1137, 5.3102) -> (-11.2807, 5.124)
  line L577 (-11.2807, 5.4909) -> (-11.4477, 5.3102)
  line L578 (-11.2807, 5.4909) -> (-11.1137, 5.3102)
  line L579 (-11.2807, 5.0132) -> (-11.1137, 4.8325)
  line L580 (-11.9645, 4.3732) -> (-11.7975, 4.187)
  line L581 (-11.6305, 4.3732) -> (-11.7975, 4.187)
  line L582 (-11.4477, 4.3732) -> (-11.2807, 4.187)
  line L583 (-11.1137, 4.3732) -> (-11.2807, 4.187)
  line L584 (-11.2807, 4.0906) -> (-11.4477, 3.9099)
  line L585 (-11.2807, 4.0906) -> (-11.1137, 3.9099)
  line L586 (-11.1137, 3.9099) -> (-11.2807, 3.7237)
  line L587 (-11.2807, 3.6252) -> (-11.4477, 3.4445)
  line L588 (-11.2807, 3.6252) -> (-11.1137, 3.4445)
  line L589 (-11.4477, 3.4445) -> (-11.2807, 3.2584)
  line L590 (-11.1137, 3.4445) -> (-11.2807, 3.2584)
  line L591 (-11.4477, 3.9099) -> (-11.2807, 3.7237)
  line L592 (-11.7975, 3.1357) -> (-11.9645, 2.955)
  line L593 (-11.7975, 3.1357) -> (-11.6305, 2.955)
  line L594 (-11.9645, 2.955) -> (-11.7975, 2.7688)
  line L595 (-11.6305, 2.955) -> (-11.7975, 2.7688)
  line L596 (-11.7975, 2.6703) -> (-11.6305, 2.4896)
  line L597 (-11.7975, 2.6703) -> (-11.9645, 2.4896)
  line L598 (-11.6305, 2.4896) -> (-11.7975, 2.3035)
  line L599 (-11.9645, 2.4896) -> (-11.7975, 2.3035)
  line L600 (-11.2807, 3.1357) -> (-11.4477, 2.955)
  line L601 (-11.2807, 3.1357) -> (-11.1137, 2.955)
  line L602 (-11.4477, 2.955) -> (-11.2807, 2.7688)
  line L603 (-11.1137, 2.955) -> (-11.2807, 2.7688)
  line L604 (-11.2807, 2.6703) -> (-11.1137, 2.4896)
  line L605 (-11.2807, 2.6703) -> (-11.4477, 2.4896)
  line L606 (-11.1137, 2.4896) -> (-11.2807, 2.3035)
  line L607 (-11.4477, 2.4896) -> (-11.2807, 2.3035)
  line L608 (-11.7975, 2.1808) -> (-11.9645, 2.0001)
  line L609 (-11.7975, 2.1808) -> (-11.6305, 2.0001)
  line L610 (-11.9645, 2.0001) -> (-11.7975, 1.8139)
  line L611 (-11.6305, 2.0001) -> (-11.7975, 1.8139)
  line L612 (-11.7975, 1.7094) -> (-11.9645, 1.5287)
  line L613 (-11.7975, 1.7094) -> (-11.6305, 1.5287)
  line L614 (-11.9645, 1.5287) -> (-11.7975, 1.3425)
  line L615 (-11.6305, 1.5287) -> (-11.7975, 1.3425)
  line L616 (-11.2807, 2.1808) -> (-11.1137, 2.0001)
  line L617 (-11.2807, 2.1808) -> (-11.4477, 2.0001)
  line L618 (-11.4477, 2.0001) -> (-11.2807, 1.8139)
  line L619 (-11.1137, 2.0001) -> (-11.2807, 1.8139)
  line L620 (-11.2807, 1.7094) -> (-11.1137, 1.5287)
  line L621 (-11.2807, 1.7094) -> (-11.4477, 1.5287)
  line L622 (-11.1137, 1.5287) -> (-11.2807, 1.3425)
  line L623 (-11.4477, 1.5287) -> (-11.2807, 1.3425)
  line L624 (-11.7975, 1.1085) -> (-11.9645, 0.9278)
  line L625 (-11.9645, 0.9278) -> (-11.7975, 0.7417)
  line L626 (-11.7975, 1.1085) -> (-11.6305, 0.9278)
  line L627 (-11.9645, 0.4502) -> (-11.7975, 0.264)
  line L628 (-11.6305, 0.4502) -> (-11.7975, 0.264)
  line L629 (-11.7975, 0.6309) -> (-11.6305, 0.4502)
  line L630 (-11.6305, 0.9278) -> (-11.7975, 0.7417)
  line L631 (-11.7975, 0.6309) -> (-11.9645, 0.4502)
  line L632 (-11.2807, 1.1085) -> (-11.4477, 0.9278)
  line L633 (-11.2807, 1.1085) -> (-11.1137, 0.9278)
  line L634 (-11.4477, 0.9278) -> (-11.2807, 0.7417)
  line L635 (-11.1137, 0.9278) -> (-11.2807, 0.7417)
  line L636 (-11.2807, 0.6309) -> (-11.1137, 0.4502)
  line L637 (-11.2807, 0.6309) -> (-11.4477, 0.4502)
  line L638 (-11.4477, 0.4502) -> (-11.2807, 0.264)
  line L639 (-11.1137, 0.4502) -> (-11.2807, 0.264)
  line L640 (-10.753, 9.764) -> (-10.92, 9.5833)
  line L641 (-10.92, 9.5833) -> (-10.753, 9.3971)
  line L642 (-10.753, 9.764) -> (-10.586, 9.5833)
  line L643 (-10.586, 9.5833) -> (-10.753, 9.3971)
  line L644 (-10.753, 9.2863) -> (-10.92, 9.1056)
  line L645 (-10.92, 9.1056) -> (-10.753, 8.9195)
  line L646 (-10.753, 9.2863) -> (-10.586, 9.1056)
  line L647 (-10.586, 9.1056) -> (-10.753, 8.9195)
  line L648 (-10.753, 8.827) -> (-10.92, 8.6463)
  line L649 (-10.92, 8.6463) -> (-10.753, 8.4602)
  line L650 (-10.753, 8.827) -> (-10.586, 8.6463)
  line L651 (-10.586, 8.6463) -> (-10.753, 8.4602)
  line L652 (-10.753, 8.3637) -> (-10.92, 8.183)
  line L653 (-10.92, 8.183) -> (-10.753, 7.9969)
  line L654 (-10.753, 8.3637) -> (-10.586, 8.183)
  line L655 (-10.586, 8.183) -> (-10.753, 7.9969)
  line L656 (-10.753, 7.8983) -> (-10.92, 7.7177)
  line L657 (-10.92, 7.7177) -> (-10.753, 7.5315)
  line L658 (-10.753, 7.8983) -> (-10.586, 7.7177)
  line L659 (-10.586, 7.7177) -> (-10.753, 7.5315)
  line L660 (-10.753, 7.4088) -> (-10.92, 7.2281)
  line L661 (-10.92, 7.2281) -> (-10.753, 7.042)
  line L662 (-10.753, 7.4088) -> (-10.586, 7.2281)
  line L663 (-10.586, 7.2281) -> (-10.753, 7.042)
  line L664 (-10.753, 6.9434) -> (-10.92, 6.7628)
  line L665 (-10.92, 6.7628) -> (-10.753, 6.5766)
  line L666 (-10.753, 6.9434) -> (-10.586, 6.7628)
  line L667 (-10.586, 6.7628) -> (-10.753, 6.5766)
  line L668 (-10.753, 6.4539) -> (-10.92, 6.2732)
  line L669 (-10.92, 6.2732) -> (-10.753, 6.0871)
  line L670 (-10.753, 6.4539) -> (-10.586, 6.2732)
  line L671 (-10.586, 6.2732) -> (-10.753, 6.0871)
  line L672 (-10.753, 5.9825) -> (-10.92, 5.8018)
  line L673 (-10.92, 5.8018) -> (-10.753, 5.6157)
  line L674 (-10.753, 5.9825) -> (-10.586, 5.8018)
  line L675 (-10.586, 5.8018) -> (-10.753, 5.6157)
  line L676 (-10.753, 5.4909) -> (-10.92, 5.3102)
  line L677 (-10.92, 5.3102) -> (-10.753, 5.124)
  line L678 (-10.753, 5.4909) -> (-10.586, 5.3102)
  line L679 (-10.753, 4.5539) -> (-10.92, 4.3732)
  line L680 (-10.753, 4.5539) -> (-10.586, 4.3732)
  line L681 (-10.92, 4.8325) -> (-10.753, 4.6463)
  line L682 (-10.586, 4.8325) -> (-10.753, 4.6463)
  line L683 (-10.753, 5.0132) -> (-10.586, 4.8325)
  line L684 (-10.586, 5.3102) -> (-10.753, 5.124)
  line L685 (-10.753, 5.0132) -> (-10.92, 4.8325)
  line L686 (-10.92, 4.3732) -> (-10.753, 4.187)
  line L687 (-10.586, 4.3732) -> (-10.753, 4.187)
  line L688 (-10.753, 4.0906) -> (-10.92, 3.9099)
  line L689 (-10.753, 4.0906) -> (-10.586, 3.9099)
  line L690 (-10.92, 3.9099) -> (-10.753, 3.7237)
  line L691 (-10.586, 3.9099) -> (-10.753, 3.7237)
  line L692 (-10.753, 3.6252) -> (-10.92, 3.4445)
  line L693 (-10.753, 3.6252) -> (-10.586, 3.4445)
  line L694 (-10.92, 3.4445) -> (-10.753, 3.2584)
  line L695 (-10.586, 3.4445) -> (-10.753, 3.2584)
  line L696 (-10.753, 3.1357) -> (-10.92, 2.955)
  line L697 (-10.753, 3.1357) -> (-10.586, 2.955)
  line L698 (-10.92, 2.955) -> (-10.753, 2.7688)
  line L699 (-10.586, 2.955) -> (-10.753, 2.7688)
  line L700 (-10.753, 2.6703) -> (-10.586, 2.4896)
  line L701 (-10.753, 2.6703) -> (-10.92, 2.4896)
  line L702 (-10.586, 2.4896) -> (-10.753, 2.3035)
  line L703 (-10.92, 2.4896) -> (-10.753, 2.3035)
  line L704 (-10.753, 2.1808) -> (-10.92, 2.0001)
  line L705 (-10.753, 2.1808) -> (-10.586, 2.0001)
  line L706 (-10.92, 2.0001) -> (-10.753, 1.8139)
  line L707 (-10.586, 2.0001) -> (-10.753, 1.8139)
  line L708 (-10.753, 1.7094) -> (-10.92, 1.5287)
  line L709 (-10.753, 1.7094) -> (-10.586, 1.5287)
  line L710 (-10.92, 1.5287) -> (-10.753, 1.3425)
  line L711 (-10.586, 1.5287) -> (-10.753, 1.3425)
  line L712 (-10.753, 1.1085) -> (-10.92, 0.9278)
  line L713 (-10.92, 0.9278) -> (-10.753, 0.7417)
  line L714 (-10.753, 1.1085) -> (-10.586, 0.9278)
  line L715 (-10.92, 0.4502) -> (-10.753, 0.264)
  line L716 (-10.586, 0.4502) -> (-10.753, 0.264)
  line L717 (-10.753, 0.6309) -> (-10.586, 0.4502)
  line L718 (-10.586, 0.9278) -> (-10.753, 0.7417)
  line L719 (-10.753, 0.6309) -> (-10.92, 0.4502)
  line L720 (-10.2362, 9.764) -> (-10.4032, 9.5833)
  line L721 (-10.4032, 9.5833) -> (-10.2362, 9.3971)
  line L722 (-10.2362, 9.764) -> (-10.0692, 9.5833)
  line L723 (-10.2362, 8.827) -> (-10.4032, 8.6463)
  line L724 (-10.2362, 8.827) -> (-10.0692, 8.6463)
  line L725 (-10.0692, 9.1056) -> (-10.2362, 8.9195)
  line L726 (-10.2362, 9.2863) -> (-10.4032, 9.1056)
  line L727 (-10.2362, 9.2863) -> (-10.0692, 9.1056)
  line L728 (-10.0692, 9.5833) -> (-10.2362, 9.3971)
  line L729 (-10.4032, 9.1056) -> (-10.2362, 8.9195)
  line L730 (-10.4032, 8.6463) -> (-10.2362, 8.4602)
  line L731 (-10.0692, 8.6463) -> (-10.2362, 8.4602)
  line L732 (-10.2362, 8.3637) -> (-10.4032, 8.183)
  line L733 (-10.2362, 8.3637) -> (-10.0692, 8.183)
  line L734 (-10.4032, 8.183) -> (-10.2362, 7.9969)
  line L735 (-10.0692, 8.183) -> (-10.2362, 7.9969)
  line L736 (-10.2362, 7.8983) -> (-10.4032, 7.7177)
  line L737 (-10.4032, 7.7177) -> (-10.2362, 7.5315)
  line L738 (-10.0692, 7.7177) -> (-10.2362, 7.5315)
  line L739 (-10.2362, 7.8983) -> (-10.0692, 7.7177)
  line L740 (-10.2362, 7.4088) -> (-10.0692, 7.2281)
  line L741 (-10.2362, 7.4088) -> (-10.4032, 7.2281)
  line L742 (-10.4032, 7.2281) -> (-10.2362, 7.042)
  line L743 (-10.0692, 7.2281) -> (-10.2362, 7.042)
  line L744 (-10.2362, 6.9434) -> (-10.0692, 6.7628)
  line L745 (-10.0692, 6.7628) -> (-10.2362, 6.5766)
  line L746 (-10.4032, 6.7628) -> (-10.2362, 6.5766)
  line L747 (-10.2362, 6.9434) -> (-10.4032, 6.7628)
  line L748 (-10.2362, 6.4539) -> (-10.4032, 6.2732)
  line L749 (-10.2362, 6.4539) -> (-10.0692, 6.2732)
  line L750 (-10.4032, 6.2732) -> (-10.2362, 6.0871)
  line L751 (-10.0692, 6.2732) -> (-10.2362, 6.0871)
  line L752 (-10.2362, 5.9825) -> (-10.4032, 5.8018)
  line L753 (-10.2362, 5.9825) -> (-10.0692, 5.8018)
  line L754 (-10.4032, 5.8018) -> (-10.2362, 5.6157)
  line L755 (-10.0692, 5.8018) -> (-10.2362, 5.6157)
  line L756 (-10.2362, 5.4909) -> (-10.4032, 5.3102)
  line L757 (-10.2362, 5.4909) -> (-10.0692, 5.3102)
  line L758 (-10.4032, 5.3102) -> (-10.2362, 5.124)
  line L759 (-10.0692, 5.3102) -> (-10.2362, 5.124)
  line L760 (-10.2362, 5.0132) -> (-10.4032, 4.8325)
  line L761 (-10.2362, 5.0132) -> (-10.0692, 4.8325)
  line L762 (-10.4032, 4.8325) -> (-10.2362, 4.6463)
  line L763 (-10.0692, 4.8325) -> (-10.2362, 4.6463)
  line L764 (-10.2362, 4.5539) -> (-10.0692, 4.3732)
  line L765 (-10.2362, 4.5539) -> (-10.4032, 4.3732)
  line L766 (-10.4032, 4.3732) -> (-10.2362, 4.187)
  line L767 (-10.0692, 4.3732) -> (-10.2362, 4.187)
  line L768 (-10.2362, 4.0906) -> (-10.4032, 3.9099)
  line L769 (-10.2362, 4.0906) -> (-10.0692, 3.9099)
  line L770 (-10.4032, 3.9099) -> (-10.2362, 3.7237)
  line L771 (-10.0692, 3.9099) -> (-10.2362, 3.7237)
  line L772 (-10.2362, 3.6252) -> (-10.4032, 3.4445)
  line L773 (-10.2362, 3.6252) -> (-10.0692, 3.4445)
  line L774 (-10.4032, 3.4445) -> (-10.2362, 3.2584)
  line L775 (-10.0692, 3.4445) -> (-10.2362, 3.2584)
  line L776 (-10.2362, 3.1357) -> (-10.4032, 2.955)
  line L777 (-10.2362, 3.1357) -> (-10.0692, 2.955)
  line L778 (-10.4032, 2.955) -> (-10.2362, 2.7688)
  line L779 (-10.0692, 2.955) -> (-10.2362, 2.7688)
  line L780 (-10.2362, 2.6703) -> (-10.0692, 2.4896)
  line L781 (-10.2362, 2.6703) -> (-10.4032, 2.4896)
  line L782 (-10.4032, 2.4896) -> (-10.2362, 2.3035)
  line L783 (-10.0692, 2.4896) -> (-10.2362, 2.3035)
  line L784 (-10.2362, 1.1085) -> (-10.4032, 0.9278)
  line L785 (-10.2362, 1.1085) -> (-10.0692, 0.9278)
  line L786 (-10.4032, 0.9278) -> (-10.2362, 0.7417)
  line L787 (-10.2362, 0.6309) -> (-10.0692, 0.4502)
  line L788 (-10.2362, 0.6309) -> (-10.4032, 0.4502)
  line L789 (-10.4032, 0.4502) -> (-10.2362, 0.264)
  line L790 (-10.0692, 0.4502) -> (-10.2362, 0.264)
  line L791 (-10.0692, 0.9278) -> (-10.2362, 0.7417)
  line L792 (-10.2362, 2.1808) -> (-10.0692, 2.0001)
  line L793 (-10.2362, 2.1808) -> (-10.4032, 2.0001)
  line L794 (-10.4032, 2.0001) -> (-10.2362, 1.8139)
  line L795 (-10.0692, 2.0001) -> (-10.2362, 1.8139)
  line L796 (-10.2362, 1.7094) -> (-10.0692, 1.5287)
  line L797 (-10.2362, 1.7094) -> (-10.4032, 1.5287)
  line L798 (-10.0692, 1.5287) -> (-10.2362, 1.3425)
  line L799 (-10.4032, 1.5287) -> (-10.2362, 1.3425)
  line L800 (-9.1525, 9.2863) -> (-9.3195, 9.1056)
  line L801 (-9.1525, 9.2863) -> (-8.9855, 9.1056)
  line L802 (-8.9855, 9.1056) -> (-9.1525, 8.9195)
  line L803 (-9.3195, 9.1056) -> (-9.1525, 8.9195)
  line L804 (-9.1525, 8.827) -> (-8.9855, 8.6463)
  line L805 (-9.1525, 8.827) -> (-9.3195, 8.6463)
  line L806 (-9.6693, 9.2863) -> (-9.5023, 9.1056)
  line L807 (-9.6693, 9.2863) -> (-9.8363, 9.1056)
  line L808 (-9.5023, 9.1056) -> (-9.6693, 8.9195)
  line L809 (-9.8363, 9.1056) -> (-9.6693, 8.9195)
  line L810 (-9.6693, 9.764) -> (-9.8363, 9.5833)
  line L811 (-9.8363, 9.5833) -> (-9.6693, 9.3971)
  line L812 (-9.5023, 9.5833) -> (-9.6693, 9.3971)
  line L813 (-9.6693, 9.764) -> (-9.5023, 9.5833)
  line L814 (-9.3195, 9.5833) -> (-9.1525, 9.3971)
  line L815 (-8.9855, 9.5833) -> (-9.1525, 9.3971)
  line L816 (-9.1525, 9.764) -> (-9.3195, 9.5833)
  line L817 (-9.1525, 9.764) -> (-8.9855, 9.5833)
  line L818 (-9.6693, 7.4088) -> (-9.8363, 7.2281)
  line L819 (-9.8363, 7.2281) -> (-9.6693, 7.042)
  line L820 (-9.6693, 6.4539) -> (-9.5023, 6.2732)
  line L821 (-9.6693, 6.4539) -> (-9.8363, 6.2732)
  line L822 (-9.5023, 6.2732) -> (-9.6693, 6.0871)
  line L823 (-9.8363, 6.2732) -> (-9.6693, 6.0871)
  line L824 (-9.1525, 5.9825) -> (-8.9855, 5.8018)
  line L825 (-9.1525, 5.9825) -> (-9.3195, 5.8018)
  line L826 (-8.9855, 5.8018) -> (-9.1525, 5.6157)
  line L827 (-9.3195, 5.8018) -> (-9.1525, 5.6157)
  line L828 (-9.6693, 5.9825) -> (-9.5023, 5.8018)
  line L829 (-9.6693, 5.9825) -> (-9.8363, 5.8018)
  line L830 (-9.5023, 5.8018) -> (-9.6693, 5.6157)
  line L831 (-9.8363, 5.8018) -> (-9.6693, 5.6157)
  line L832 (-9.3195, 4.8325) -> (-9.1525, 4.6463)
  line L833 (-8.9855, 4.8325) -> (-9.1525, 4.6463)
  line L834 (-9.6693, 5.0132) -> (-9.5023, 4.8325)
  line L835 (-9.6693, 5.0132) -> (-9.8363, 4.8325)
  line L836 (-9.1525, 4.5539) -> (-8.9855, 4.3732)
  line L837 (-9.1525, 4.5539) -> (-9.3195, 4.3732)
  line L838 (-9.5023, 4.8325) -> (-9.6693, 4.6463)
  line L839 (-9.8363, 4.8325) -> (-9.6693, 4.6463)
  line L840 (-9.6693, 4.5539) -> (-9.5023, 4.3732)
  line L841 (-9.6693, 4.5539) -> (-9.8363, 4.3732)
  line L842 (-9.5023, 3.4445) -> (-9.6693, 3.2584)
  line L843 (-9.8363, 3.4445) -> (-9.6693, 3.2584)
  line L844 (-9.6693, 3.6252) -> (-9.5023, 3.4445)
  line L845 (-9.6693, 3.6252) -> (-9.8363, 3.4445)
  line L846 (-9.8363, 3.9099) -> (-9.6693, 3.7237)
  line L847 (-9.6693, 4.0906) -> (-9.5023, 3.9099)
  line L848 (-9.6693, 4.0906) -> (-9.8363, 3.9099)
  line L849 (-9.5023, 3.9099) -> (-9.6693, 3.7237)
  line L850 (-9.6693, 8.827) -> (-9.8363, 8.6463)
  line L851 (-9.8363, 8.6463) -> (-9.6693, 8.4602)
  line L852 (-9.6693, 8.827) -> (-9.5023, 8.6463)
  line L853 (-9.5023, 8.6463) -> (-9.6693, 8.4602)
  line L854 (-9.6693, 8.3637) -> (-9.8363, 8.183)
  line L855 (-9.8363, 8.183) -> (-9.6693, 7.9969)
  line L856 (-9.6693, 8.3637) -> (-9.5023, 8.183)
  line L857 (-8.9855, 8.6463) -> (-9.1525, 8.4602)
  line L858 (-9.3195, 8.6463) -> (-9.1525, 8.4602)
  line L859 (-9.1525, 8.3637) -> (-8.9855, 8.183)
  line L860 (-8.9855, 8.183) -> (-9.1525, 7.9969)
  line L861 (-9.3195, 8.183) -> (-9.1525, 7.9969)
  line L862 (-9.5023, 8.183) -> (-9.6693, 7.9969)
  line L863 (-9.1525, 8.3637) -> (-9.3195, 8.183)
  line L864 (-9.6693, 7.8983) -> (-9.8363, 7.7177)
  line L865 (-9.8363, 7.7177) -> (-9.6693, 7.5315)
  line L866 (-9.6693, 7.4088) -> (-9.5023, 7.2281)
  line L867 (-9.5023, 7.2281) -> (-9.6693, 7.042)
  line L868 (-9.5023, 7.7177) -> (-9.6693, 7.5315)
  line L869 (-9.6693, 7.8983) -> (-9.5023, 7.7177)
  line L870 (-9.1525, 6.9434) -> (-9.3195, 6.7628)
  line L871 (-9.1525, 6.9434) -> (-8.9855, 6.7628)
  line L872 (-9.1525, 7.4088) -> (-9.3195, 7.2281)
  line L873 (-8.9855, 7.2281) -> (-9.1525, 7.042)
  line L874 (-9.3195, 7.7177) -> (-9.1525, 7.5315)
  line L875 (-9.1525, 7.8983) -> (-9.3195, 7.7177)
  line L876 (-9.1525, 7.8983) -> (-8.9855, 7.7177)
  line L877 (-8.9855, 7.7177) -> (-9.1525, 7.5315)
  line L878 (-9.1525, 7.4088) -> (-8.9855, 7.2281)
  line L879 (-9.3195, 7.2281) -> (-9.1525, 7.042)
  line L880 (-9.6693, 6.9434) -> (-9.8363, 6.7628)
  line L881 (-9.8363, 6.7628) -> (-9.6693, 6.5766)
  line L882 (-9.6693, 6.9434) -> (-9.5023, 6.7628)
  line L883 (-9.5023, 6.7628) -> (-9.6693, 6.5766)
  line L884 (-9.3195, 6.2732) -> (-9.1525, 6.0871)
  line L885 (-8.9855, 6.2732) -> (-9.1525, 6.0871)
  line L886 (-9.1525, 6.4539) -> (-9.3195, 6.2732)
  line L887 (-9.1525, 6.4539) -> (-8.9855, 6.2732)
  line L888 (-9.3195, 6.7628) -> (-9.1525, 6.5766)
  line L889 (-8.9855, 6.7628) -> (-9.1525, 6.5766)
  line L890 (-9.6693, 5.4909) -> (-9.8363, 5.3102)
  line L891 (-9.8363, 5.3102) -> (-9.6693, 5.124)
  line L892 (-9.6693, 5.4909) -> (-9.5023, 5.3102)
  line L893 (-9.1525, 5.0132) -> (-9.3195, 4.8325)
  line L894 (-9.5023, 5.3102) -> (-9.6693, 5.124)
  line L895 (-9.3195, 5.3102) -> (-9.1525, 5.124)
  line L896 (-8.9855, 5.3102) -> (-9.1525, 5.124)
  line L897 (-9.1525, 5.4909) -> (-9.3195, 5.3102)
  line L898 (-9.1525, 5.4909) -> (-8.9855, 5.3102)
  line L899 (-9.1525, 5.0132) -> (-8.9855, 4.8325)
  line L900 (-9.8363, 4.3732) -> (-9.6693, 4.187)
  line L901 (-9.5023, 4.3732) -> (-9.6693, 4.187)
  line L902 (-9.3195, 4.3732) -> (-9.1525, 4.187)
  line L903 (-8.9855, 4.3732) -> (-9.1525, 4.187)
  line L904 (-9.1525, 4.0906) -> (-9.3195, 3.9099)
  line L905 (-9.1525, 4.0906) -> (-8.9855, 3.9099)
  line L906 (-8.9855, 3.9099) -> (-9.1525, 3.7237)
  line L907 (-9.1525, 3.6252) -> (-9.3195, 3.4445)
  line L908 (-9.1525, 3.6252) -> (-8.9855, 3.4445)
  line L909 (-9.3195, 3.4445) -> (-9.1525, 3.2584)
  line L910 (-8.9855, 3.4445) -> (-9.1525, 3.2584)
  line L911 (-9.3195, 3.9099) -> (-9.1525, 3.7237)
  line L912 (-9.6693, 3.1357) -> (-9.8363, 2.955)
  line L913 (-9.6693, 3.1357) -> (-9.5023, 2.955)
  line L914 (-9.8363, 2.955) -> (-9.6693, 2.7688)
  line L915 (-9.5023, 2.955) -> (-9.6693, 2.7688)
  line L916 (-9.6693, 2.6703) -> (-9.5023, 2.4896)
  line L917 (-9.6693, 2.6703) -> (-9.8363, 2.4896)
  line L918 (-9.5023, 2.4896) -> (-9.6693, 2.3035)
  line L919 (-9.8363, 2.4896) -> (-9.6693, 2.3035)